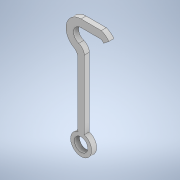
# Autodesk Inventor part: Hook
Saved by Autodesk Inventor 2022 (Build 260153000, 153)
## iProperties
Created: 2023-02-27
Part Number: Hook
Material: Generic
Document SubType Name: Modeling
Designer: zarek
Density: 1 g/cm^3
Appearance: Default
Author: zarek
Autodesk Inventor part; units mm, degrees
ref_plane "YZ Plane" through (0, 0, 0) normal (1, 0, 0) x (0, 1, 0)
ref_plane "XZ Plane" through (0, 0, 0) normal (0, 1, 0) x (-1, 0, 0)
ref_plane "XY Plane" through (0, 0, 0) normal (0, 0, 1) x (1, 0, 0)
sketch "Sketch1" plane through (0, 0, 0) normal (0, 0, 1) x (1, 0, 0)
  circle A0 centre (0, 0) radius 2.667
  circle A1 centre (0, 0) radius 4.167
  line L0 (-1.25, 3.9751) -> (1.25, 3.9751)
  line L1 (1.25, 3.9751) -> (1.25, 37.2251)
  line L2 (1.25, 37.2251) -> (-1.25, 37.2251)
  line L3 (-1.25, 37.2251) -> (-1.25, 3.9751)
  line L4 (0, 0) -> (0, 14.9208)
  circle A2 centre (0, 37.2251) radius 3
  circle A3 centre (0, 37.2251) radius 6
  line L5 (0, 43.2251) -> (8, 43.2251)
  line L6 (8, 43.2251) -> (8, 40.2251)
  line L7 (8, 40.2251) -> (0, 40.2251)
  circle A4 centre (6, 37.2251) radius 6.3246
  circle A5 centre (6, 37.2251) radius 3.6056
  line L8 (8.94, 39.3122) -> (11.0685, 41.008)
  point P0 (-1.25, 31.3567)
  point P1 (1.25, 3.9751)
  point P2 (1.25, 3.9751)
  point P3 (1.25, 34.4979)
  dimension "d1" = 8.334
  dimension "d5" = 6
  dimension "d0" = 5.334
  dimension "d2" = 1.25
  dimension "d3" = 1.25
  dimension "d4" = 33.25
  dimension "d6" = 12
  dimension "d7" = 8
  constraints: 18 end point, 6 point on circle, 4 centre point, 4 coincident, 3 horizontal, 2 parallel, 2 perpendicular, 1 midpoint, 1 point on line, 1 tangent, 1 vertical, 6 other
  measures "d0" diameter of A0
  measures "d2" distance between parallel lines of L3 L4
  measures "d3" distance between parallel lines of L1 L4
  measures "d4" distance between parallel lines of L0 L2
  measures "d6" diameter of A3
  measures "d7" distance from line of L6 L5.start
extrude "Extrusion1" add sketch "Sketch1" along normal blind 2 contours L0 A1 | L0 A1 L4 | L4 A1 L0 | L3 A3 L1 A1 | A3 A4 L7 A2 L3 | L3 A2 A4 L1 A3 | L5 A4 A3 | A4 A2 L1 | A4 L5 L6 A5 A3 | A3 A5 L7 A4 | A5 L7 A3 | A3 L7 A5 | A4 L8 A5 L6 picked at (6.8274, 40.3479) picked at (4.4958, 40.2834)
fillet "Fillet1" radius 3.175 2 edges at (1.25, 34.4979, 1) (-1.25, 31.3567, 1)
equation "\"d2\" = d3"
body "Solid1"
